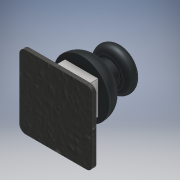
# Autodesk Inventor part: JoyStick
Saved by Autodesk Inventor 2018 (Build 220112000, 112)
## iProperties
Created: 2019-10-10
Part Number: JoyStick
Material: Типовые
Document SubType Name: Modeling
Designer: Professional
Density: 1 g/cm^3
Appearance: По умолчанию
Author: Professional
Autodesk Inventor part; units mm, degrees
ref_plane "YZ Plane" through (0, 0, 0) normal (1, 0, 0) x (0, 1, 0)
ref_plane "XZ Plane" through (0, 0, 0) normal (0, 1, 0) x (-1, 0, 0)
ref_plane "XY Plane" through (0, 0, 0) normal (0, 0, 1) x (1, 0, 0)
sketch "Эскиз1" plane through (0, 0, 0) normal (0, 1, 0) x (-1, 0, 0)
  line L0 (17.6, 17.6) -> (-17.6, 17.6)
  line L1 (-17.6, 17.6) -> (-17.6, -17.6)
  line L2 (-17.6, -17.6) -> (17.6, -17.6)
  line L3 (17.6, -17.6) -> (17.6, 17.6)
  point P0 (0, 0)
  dimension "d0" = 35.2
  dimension "d1" = 35.2
  dimension "d2" = 17.6
  dimension "d3" = 17.6
  constraints: 8 end point, 2 parallel, 1 horizontal, 1 perpendicular
  measures "d0" distance between parallel lines of L2 L0
  measures "d1" distance of L1.end L2.end
  measures "d2" distance from line of point (0, 0) L0
  measures "d3" distance from line of point (0, 0) L3
extrude "Выдавливание1" add sketch "Эскиз1" along normal blind 1.8
fillet "Сопряжение1" radius 3 4 edges at (17.6, 0.9, 17.6) (-17.6, 0.9, 17.6) (17.6, 0.9, -17.6) (-17.6, 0.9, -17.6)
sketch "Эскиз2" plane through (0, 1.8, 0) normal (0, 1, 0) x (1, 0, 0)
  line L0 (-9.4, -9.4) -> (6.6, -9.4)
  line L1 (6.6, -9.4) -> (6.6, 6.6)
  line L2 (6.6, 6.6) -> (-9.4, 6.6)
  line L3 (-9.4, 6.6) -> (-9.4, -9.4)
  line L4 (-14.6, -17.6) -> (14.6, -17.6) projected
  line L5 (-17.6, 14.6) -> (-17.6, -14.6) projected
  point P0 (0, 0)
  dimension "d7" = 16
  dimension "d8" = 16
  dimension "d9" = 8.2
  dimension "d10" = 8.2
  constraints: 8 end point, 2 parallel, 1 horizontal, 1 perpendicular
  measures "d7" distance of L0.start L0.end
  measures "d8" distance of L0.end L1.end
  measures "d9" distance between parallel lines of L4 L0
  measures "d10" distance between parallel lines of L5 L3
extrude "Выдавливание2" add sketch "Эскиз2" along normal blind 12
sketch "Эскиз3" plane through (0, 1.8, 0) normal (0, 1, 0) x (1, 0, 0)
  line L0 (14.1, -12.6) -> (15.6, -12.6)
  line L1 (15.6, -12.6) -> (15.6, 12.6)
  line L2 (15.6, 12.6) -> (14.1, 12.6)
  line L3 (14.1, 12.6) -> (14.1, -12.6)
  line L4 (-14.6, -17.6) -> (14.6, -17.6) projected
  line L5 (14.6, 17.6) -> (-14.6, 17.6) projected
  line L6 (17.6, -14.6) -> (17.6, 14.6) projected
  point P0 (0, 0)
  dimension "d13" = 5
  dimension "d14" = 5
  dimension "d15" = 2
  dimension "d16" = 1.5
  constraints: 8 end point, 2 parallel, 1 horizontal, 1 perpendicular
  measures "d13" distance between parallel lines of L4 L0
  measures "d14" distance between parallel lines of L5 L2
  measures "d15" distance between parallel lines of L6 L1
  measures "d16" distance between parallel lines of L1 L3
extrude "Выдавливание3" add sketch "Эскиз3" along normal blind 0.1
sketch "Эскиз4" plane through (0, 13.8, 0) normal (0, 1, 0) x (1, 0, 0)
  circle A0 centre (-1.4, -1.4) radius 5.5
  line L0 (-9.4, 6.6) -> (-9.4, -9.4) projected
  line L1 (-9.4, -9.4) -> (6.6, -9.4) projected
  point P0 (0, 0)
  dimension "d19" = 11
  dimension "d20" = 8
  dimension "d21" = 8
  constraints: 1 centre point
  measures "d19" diameter of A0
  measures "d20" distance from line of L0 A0.centre
  measures "d21" distance from line of L1 A0.centre
extrude "Выдавливание4" add sketch "Эскиз4" along normal blind 19
sketch "Эскиз5" plane through (0, 13.8, 0) normal (0, 1, 0) x (1, 0, 0)
  circle A0 centre (-1.4, -1.4) radius 5.5 projected
  circle A1 centre (-1.4, -1.4) radius 13.5
  point P0 (0, 0)
  dimension "d24" = 27
  constraints: 1 centre point, 1 coincident
  measures "d24" diameter of A1
extrude "Выдавливание5" add sketch "Эскиз5" along normal blind 8.5
fillet "Сопряжение2" radius 8 1 edges at (-14.9, 22.3, 1.4)
sketch "Эскиз6" plane through (-1.4, 32.8, 1.4) normal (0, 1, 0) x (1, 0, 0)
  circle A0 centre (0, 0) radius 5.5 projected
  circle A1 centre (0, 0) radius 10
  point P0 (1.4, 1.4)
  dimension "d28" = 20
  constraints: 1 centre point, 1 coincident
  measures "d28" diameter of A1
extrude "Выдавливание6" add sketch "Эскиз6" against normal blind 6
full round fillet "Сопряжение3" first side at (-0.4307, 32.8, 1.4) centre faces at (8.4705, 28.8, 3.0041) second side at (6.9499, 26.8, 2.6365)
